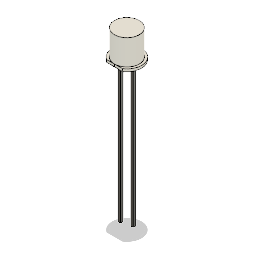
2831 Photo Transistor Light Sensor (Autodesk Fusion 360 design; units mm, degrees)
Autodesk Fusion 360 part; units mm, degrees
note: some values were not read from the file. Chosen so that the rebuilt part matches the saved one: which face or edge a step refers to. Set by a fixed rule: which sketch regions a step uses.
sketch "Sketch1" plane through (0, 0, 0) normal (0, 1, 0) x (1, 0, 0)
  circle A0 centre (0, 0) radius 2.45
  line L0 (5, -2.45) -> (-5, -2.45) construction
  arc A1 (1.5516, -2.45) -> (-1.5516, -2.45) centre (0, 0) ccw
  line L1 (-1.5516, -2.45) -> (1.5516, -2.45)
  line L2 (0, 8) -> (0, -8) construction
  line L3 (8, 0) -> (-8, 0) construction
  line L4 (0.25, -1.5) -> (-0.25, -1.5)
  line L5 (-0.25, -1.5) -> (-0.25, -1)
  line L6 (-0.25, -1) -> (0.25, -1)
  line L7 (0.25, -1) -> (0.25, -1.5)
  line L8 (0.25, -1.5) -> (-0.25, -1) construction
  line L9 (-0.25, -1.5) -> (0.25, -1) construction
  line L10 (-0.25, 1) -> (0.25, 1)
  line L11 (-0.25, 1.5) -> (-0.25, 1)
  line L12 (0.25, 1.5) -> (-0.25, 1.5)
  line L13 (0.25, 1) -> (0.25, 1.5)
  line L14 (-0.25, 1.5) -> (0.25, 1) construction
  line L15 (0.25, 1.5) -> (-0.25, 1) construction
  point P0 (0, -20)
  point P1 (0, -20)
  dimension "d7" = 5.8
  dimension "d8" = 4.9
  dimension "d22" = 16
  dimension "d23" = 16
  dimension "d24" = 0.5
  dimension "d25" = 0.5
  dimension "d26" = 1.25
  measures "d7" diameter of A1
  measures "d8" diameter of A0
  measures "d25" distance of A0.centre
extrude "Extrude4" add sketch "Sketch1" against normal blind 29 contours L10 L11 L12 L13 makes body 1
extrude "Extrude3" add sketch "Sketch1" against normal blind 27 separate body contours L4 L5 L6 L7 makes body 2
extrude "Extrude2" add sketch "Sketch1" along normal blind 0.5 separate body contours A1 L1 makes body 3
extrude "Extrude1" add sketch "Sketch1" along normal blind 5.5 separate body contours A0 | L4 L5 L6 L7 | L10 L11 L12 L13 makes body 4
copy_body "CutPasteBodies1" bodies 3 4 removing the originals makes body 5 makes body 6 in component "Sensor"
copy_body "CutPasteBodies1'" bodies 1 2 removing the originals makes body 7 makes body 8 in component "Leads"
component "Sensor" placed x (1, 0, 0) y (0, 1, 0) z (0, 0, 1) at (0, 0, 0)
component "Leads" placed x (1, 0, 0) y (0, 1, 0) z (0, 0, 1) at (0, 0, 0)
equation "SensorHeight = 5.5 mm"
equation "SensorDiameter = 4.9 mm" comment "The cylinder, not the base flange."
equation "BaseDiameter = 5.8 mm"
equation "EmitterLeadLength = 27 mm"
equation "CollectorLeadLength = EmitterLeadLength + 2 mm"
equation "LeadSpacing = 2.5 mm"
equation "d7 = BaseDiameter"
equation "d8 = SensorDiameter"
equation "LeadThickness = 0.5 mm"
equation "d17 = SensorHeight"
equation "BaseHeight = 0.5 mm"
equation "d20 = BaseHeight"
equation "d24 = LeadThickness"
equation "d25 = LeadThickness"
equation "d26 = LeadSpacing / 2"
equation "d27 = -EmitterLeadLength"
equation "d29 = -CollectorLeadLength"
named bodies: "Sensor", "Base", "Emitter", "Collector"
